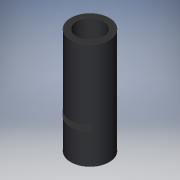
# Autodesk Inventor part: Housing
Saved by Autodesk Inventor 2018 (Build 220112000, 112)
## iProperties
Created: 2019-07-12
Part Number: Housing
Material: Generic
Document SubType Name: Modeling
Designer: aal_9
Density: 1 g/cm^3
Appearance: Default
Author: aal_9
Autodesk Inventor part; units mm, degrees
ref_plane "YZ Plane" through (0, 0, 0) normal (1, 0, 0) x (0, 1, 0)
ref_plane "XY Plane" through (0, 0, 0) normal (0, 0, 1) x (1, 0, 0)
sketch "Sketch1" plane through (0, 0, 0) normal (0, 0, 1) x (1, 0, 0)
  circle A0 centre (0, 0) radius 20
  dimension "d0" = 40
  constraints: 1 centre point, 1 coincident
  measures "d0" diameter of A0
extrude "Extrusion1" add sketch "Sketch1" along normal blind 110
ref_plane "Work Plane2" through (0, 20, 0) normal (0, 1, 0) x (-1, 0, 0)
sketch "Sketch3" plane through (0, 20, 0) normal (0, 1, 0) x (-1, 0, 0)
  circle A0 centre (0, 54) radius 7
  circle A1 centre (0, 71.5) radius 7
  point P0 (0, 0)
  dimension "d3" = 14
  dimension "d4" = 14
  dimension "d5" = 17.5
  dimension "d6" = 54
  dimension "d7" = 0
  dimension "d8" = 0
  constraints: 2 centre point
  measures "d3" diameter of A1
  measures "d4" diameter of A0
  measures "d5" distance of A0.centre A1.centre
  measures "d6" distance of point (0, 0) A0.centre
  measures "d7" horizontal distance of point (0, 0) A1.centre
  measures "d8" horizontal distance of point (0, 0) A0.centre
extrude "Extrusion2" cut sketch "Sketch3" against normal blind 4
sketch "Sketch4" plane through (0, 16, 71.5) normal (0, 1, 0) x (1, 0, 0)
  circle A0 centre (0, 0) radius 7 projected
  circle A1 centre (0, 0) radius 5.9531
  circle A2 centre (0, 17.5) radius 7 projected
  circle A3 centre (0, 17.5) radius 5.9531
  point P0 (0, 71.5)
  dimension "d11" = 11.9062
  dimension "d12" = 11.9062
  constraints: 2 centre point, 2 coincident
  measures "d11" diameter of A1
  measures "d12" diameter of A3
extrude "Extrusion3" cut sketch "Sketch4" against normal blind 23 contours A1 | A3
sketch "Sketch5" plane through (0, 0, 0) normal (0, 0, -1) x (-1, 0, 0)
  circle A0 centre (0, -7) radius 11.125
  point P0 (0, 0)
  dimension "d15" = 22.25
  dimension "d40" = 0
  dimension "d63" = 7
  constraints: 1 centre point
  measures "d15" diameter of A0
  measures "d40" horizontal distance of A0.centre point (0, 0)
  measures "d63" distance of A0.centre point (0, 0)
extrude "Extrusion4" cut sketch "Sketch5" against normal blind 15
sketch "Sketch6" plane through (0, -7, 15) normal (0, 0, -1) x (-1, 0, 0)
  circle A0 centre (0, 0) radius 5.85
  circle A1 centre (0, 0) radius 11.125 projected
  point P0 (0, 7)
  dimension "d19" = 11.7
  constraints: 1 centre point, 1 concentric
  measures "d19" diameter of A0
extrude "Extrusion5" cut sketch "Sketch6" against normal blind 0.3 contours A0
sketch "Sketch7" plane through (0, -7, 15.3) normal (0, 0, -1) x (-1, 0, 0)
  circle A0 centre (0, 0) radius 5
  circle A1 centre (0, 0) radius 5.85 projected
  point P0 (0, 7)
  dimension "d22" = 10
  constraints: 1 centre point, 1 concentric
  measures "d22" diameter of A0
extrude "Extrusion6" cut sketch "Sketch7" against normal blind 9 contours A0
sketch "Sketch8" plane through (0, -7, 24.3) normal (0, 0, -1) x (-1, 0, 0)
  circle A0 centre (0, 0) radius 3.5
  circle A1 centre (0, 0) radius 5 projected
  point P0 (0, 7)
  dimension "d25" = 7
  constraints: 1 centre point, 1 concentric
  measures "d25" diameter of A0
extrude "Extrusion7" cut sketch "Sketch8" against normal blind 18 contours A0
sketch "Sketch9" plane through (0, -7, 15) normal (0, 0, -1) x (-1, 0, 0)
  circle A0 centre (-7.4, 0) radius 1.25
  circle A1 centre (0, 0) radius 3.5 projected
  point P0 (0, 7)
  dimension "d28" = 2.5
  dimension "d29" = 7.4
  dimension "d30" = 0
  constraints: 1 centre point
  measures "d28" diameter of A0
  measures "d29" distance of A1.centre A0.centre
  measures "d30" vertical distance of A1.centre A0.centre
extrude "Extrusion8" cut sketch "Sketch9" against normal blind 2 contours A0
ref_plane "Work Plane3" through (0, -7, 34.3) normal (0, 0, -1) x (-1, 0, 0)
sketch "Sketch11" plane through (0, -7, 34.3) normal (0, 0, -1) x (-1, 0, 0)
  circle A0 centre (0, 0) radius 3.5 projected
  circle A1 centre (0, 0) radius 16
  point P0 (0, 7)
  dimension "d37" = 32
  constraints: 1 centre point, 1 coincident
  measures "d37" diameter of A1
extrude "Extrusion10" cut sketch "Sketch11" along normal mid plane 5.5
sketch "Sketch12" plane through (0, 0, 0) normal (0, 0, -1) x (-1, 0, 0)
  circle A0 centre (-9, 9) radius 3
  circle A1 centre (0, 0) radius 20 projected
  dimension "d58" = 6
  dimension "d59" = 9
  dimension "d60" = 9
  constraints: 1 centre point
  measures "d58" diameter of A0
  measures "d59" horizontal distance of A1.centre A0.centre
  measures "d60" horizontal distance of A1.centre A0.centre
sketch "Sketch13" plane through (0, 0, 110) normal (0, 0, 1) x (1, 0, 0)
  circle A0 centre (0, 0) radius 14
  dimension "d44" = 28
  constraints: 1 centre point, 1 coincident
  measures "d44" diameter of A0
extrude "Extrusion11" cut sketch "Sketch13" against normal blind 65
ref_plane "Work Plane5" through (0, 13, 71.5) normal (0, 1, 0) x (1, 0, 0)
sketch "Sketch15" plane through (0, 13, 71.5) normal (0, 1, 0) x (1, 0, 0)
  circle A0 centre (0, 17.5) radius 7 projected
  circle A1 centre (0, 17.5) radius 8.5
  circle A2 centre (0, 0) radius 7 projected
  circle A3 centre (0, 0) radius 8.5
  point P0 (0, 71.5)
  dimension "d54" = 17
  dimension "d55" = 17
  constraints: 2 centre point, 2 coincident
  measures "d54" diameter of A1
  measures "d55" diameter of A3
extrude "Extrusion14" cut sketch "Sketch15" against normal blind 10 contours A0 | A2
extrude "Extrusion15" cut sketch "Sketch12" against normal up to surface (45 mm away) contours A0
body "Solid1"
